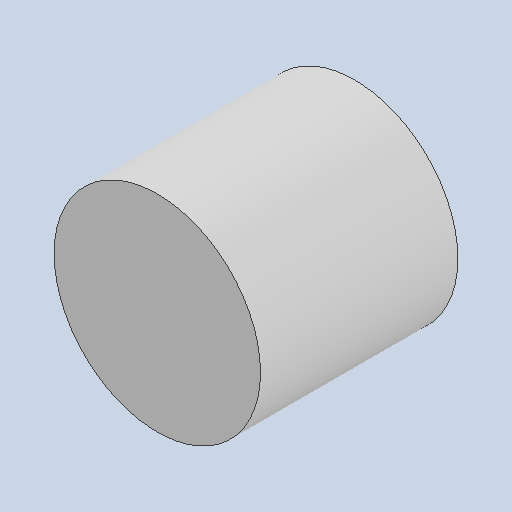
# Autodesk Inventor part: opona
Saved by Autodesk Inventor 2023 (Build 270158000, 158)
## iProperties
Created: 2022-12-08
Part Number: opona
Material: Generic
Document SubType Name: Modeling
Designer: Kamil
Density: 1 g/cm^3
Appearance: Default
Author: Kamil
Autodesk Inventor part; units mm, degrees
ref_plane "YZ Plane" through (0, 0, 0) normal (1, 0, 0) x (0, 1, 0)
ref_plane "XZ Plane" through (0, 0, 0) normal (0, 1, 0) x (-1, 0, 0)
ref_plane "XY Plane" through (0, 0, 0) normal (0, 0, 1) x (1, 0, 0)
sketch "Sketch1" plane through (0, 0, 0) normal (0, 0, 1) x (1, 0, 0)
  circle A0 centre (0, 0) radius 13.1 projected
  line L0 (0, 0) -> (-8.5876, 9.8926)
  line L1 (-8.5876, 9.8926) -> (-10.5542, 12.1581)
  circle A1 centre (0, 0) radius 16.1
  point P0 (0, 0)
  dimension "d0" = 3
  constraints: 4 end point, 1 coincident, 5 other
  measures "d0" distance of L0.end L1.end
extrude "Extrusion1" add sketch "Sketch1" against normal blind 28.2
sketch "Sketch2" plane through (0, 0, 0) normal (0, 0, 1) x (1, 0, 0)
  circle A0 centre (0, 0) radius 13.1 projected
  point P0 (0, 0)
extrude "Extrusion2" add sketch "Sketch2" against normal blind 2.85
sketch "Sketch4" plane through (0, 0, -28.2) normal (0, 0, -1) x (-1, 0, 0)
  circle A0 centre (0, 0) radius 16.1 projected
  circle A1 centre (0, 0) radius 13.1 projected
  circle A2 centre (0, 0) radius 12.5
  point P0 (0, 0)
  constraints: 1 centre point, 2 other
extrude "Extrusion3" add sketch "Sketch4" along normal blind 2.6 contours A0 | A1
body "Solid1"
